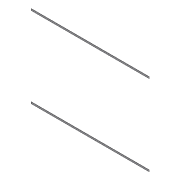
# Autodesk Inventor part: Tape_key
Saved by Autodesk Inventor 2012 (Build 160160000, 160)
## iProperties
Created: 2011-07-01
Part Number: Tape_key
Document SubType Name: Modeling
Designer: dfoster
Density: 1 g/cm^3
Material: Default
Author: dfoster
Autodesk Inventor part; units mm, degrees
ref_plane "YZ Plane" through (0, 0, 0) normal (1, 0, 0) x (0, 1, 0)
ref_plane "XZ Plane" through (0, 0, 0) normal (0, 1, 0) x (-1, 0, 0)
ref_plane "XY Plane" through (0, 0, 0) normal (0, 0, 1) x (1, 0, 0)
sketch "Sketch1" plane through (0, 0, 0) normal (0, 0, 1) x (1, 0, 0)
  line L0 (0, 0) -> (3683, 0)
  line L1 (3683, 0) -> (3683, 50.8)
  line L2 (3683, 50.8) -> (0, 50.8)
  line L3 (0, 50.8) -> (0, 0)
  dimension "d0" = 50.8
  dimension "d1" = 3683
  constraints: 8 end point, 2 parallel, 1 horizontal, 1 perpendicular
  measures "d0" distance between parallel lines of L0 L2
  measures "d1" distance of L0.start L0.end
extrude "Extrusion1" add sketch "Sketch1" along normal blind 4.7752
pattern_linear "Rectangular Pattern1" count 2 spacing 2514.6 along (0, 1, 0) of "Extrusion1"
body "Solid1"
